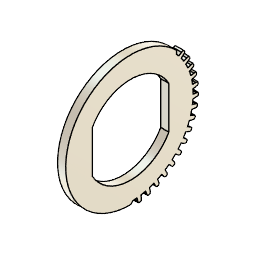
Gear_ (Autodesk Fusion 360 design; units mm, degrees)
Autodesk Fusion 360 part; units mm, degrees
sketch "Sketch1" plane through (0, 0, 0) normal (1, 0, 0) x (0, 1, 0)
  line L0 (-14, 7.746) -> (-14, -7.746)
  line L1 (14, -7.746) -> (14, 7.746)
  line L2 (0, 0) -> (0, 30.2965) construction
  arc A0 (-14, -7.746) -> (14, -7.746) centre (0, 0) ccw
  arc A1 (14, 7.746) -> (-14, 7.746) centre (0, 0) ccw
  line L3 (16.8429, 16.8154) -> (16.8429, 15.5154)
  line L4 (0.0194, -23.8) -> (0.9387, -22.8808)
  arc A2 (16.8429, 16.8154) -> (0.0194, -23.8) centre (0, 0) ccw
  arc A3 (0.9387, -22.8808) -> (16.8429, 15.5154) centre (0, 0) ccw
  dimension "d1" = 47.6
  dimension "d2" = 32
  dimension "d3" = 28
  dimension "d4" = 45.8
  dimension "d5" = 135
  dimension "d6" = 1.3
  dimension "d7" = 1.3
  constraint coincident L2.start A0.centre
  constraint concentric A0 A2
  constraint vertical L0
  constraint coincident L1.end A0
  constraint parallel L0 L1
  constraint parallel L1 L2
  constraint symmetric L0 L1 L2
  constraint concentric A0 A1
  constraint vertical L3
  measures "d1" diameter of A2
  measures "d2" diameter of A0
  measures "d3" distance of L0 L1
  measures "d4" diameter of A3
  measures "d5" angle of L3 L4
  measures "d6" distance of L4.start L4.end
  measures "d7" distance of L3.start L3.end
extrude "Extrude1" add sketch "Sketch1" along normal blind 3
sketch "Sketch2" plane through (3, 0, 0) normal (1, 0, 0) x (0, 1, 0)
  arc A0 (14, 7.746) -> (-14, 7.746) centre (0, 0) ccw
  line L0 (14, 7.746) -> (14, -7.746)
  arc A1 (-14, -7.746) -> (14, -7.746) centre (0, 0) ccw
  line L1 (-14, -7.746) -> (-14, 7.746)
  arc A2 (16.8429, 16.8154) -> (0.0194, -23.8) centre (0, 0) ccw
  line L2 (0.0194, -23.8) -> (0.9387, -22.8808)
  arc A3 (0.9387, -22.8808) -> (16.8429, 15.5154) centre (0, 0) ccw
  line L3 (16.8429, 15.5154) -> (16.8429, 16.8154)
  line L4 (0, 0) -> (32.1047, 24.8771) construction
  line L5 (17.6325, 14.6118) -> (18.628, 15.2818)
  arc A4 (19.3793, 15.5858) -> (18.628, 15.2818) centre (19.7243, 13.653) ccw
  line L6 (19.3793, 15.5858) -> (19.6549, 15.2301)
  line L7 (18.5513, 13.4261) -> (19.4486, 14.2228)
  arc A5 (19.4486, 14.2228) -> (19.9306, 14.8744) centre (18.1451, 15.691) ccw
  line L8 (19.9306, 14.8744) -> (19.6549, 15.2301)
  dimension "d10" = 1.2
  dimension "d11" = 1.2
  dimension "d12" = 2
  dimension "d13" = 0.45
  dimension "d14" = 0.75
  constraint coincident A0.centre A1.centre
  constraint coincident A3 L5.start
  constraint tangent L5 A4
  constraint coincident L4 L6.end
  constraint perpendicular L4 L6
  constraint symmetric L4 L5.start L7.start
  constraint symmetric L4 L5.end L7.end
  constraint symmetric L4 A4.start A5.end
  constraint symmetric L4 A4 A5
  constraint symmetric L4 L6.end L8.end
  measures "d10" distance of A3.end L5.start
  measures "d11" distance of L5.start L5.end
  measures "d12" distance of L5.start A4.start
  measures "d13" distance of L4 A4.start
  measures "d14" distance of L4 L5.start
extrude "Extrude2" add sketch "Sketch2" against normal blind 3 contours A3 L5 A4 L6 L7 A5 L8
pattern_circular "C-Pattern1" count 16 over 120 about axis through (0, 0, 0) along (-1, 0, 0) of "Extrude2"
